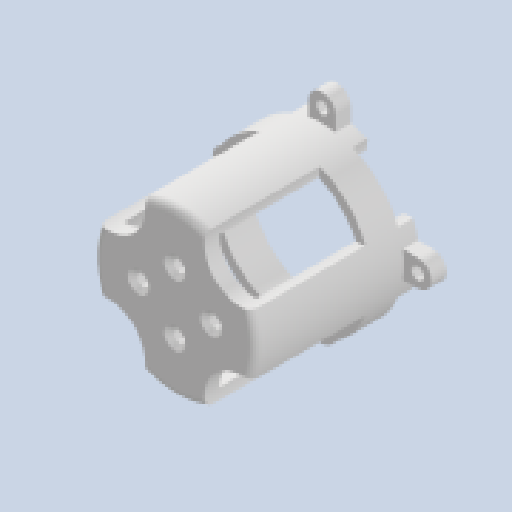
# Autodesk Inventor part: Capac_MOTOR
Saved by Autodesk Inventor 2024 (Build 280153000, 153)
## iProperties
Created: 2024-04-22
Part Number: Capac_MOTOR
Material: Generic
Document SubType Name: Modeling
Designer: mirun
Density: 1 g/cm^3
Appearance: Default
Author: mirun
Autodesk Inventor part; units mm, degrees
ref_plane "YZ Plane" through (0, 0, 0) normal (1, 0, 0) x (0, 1, 0)
ref_plane "XZ Plane" through (0, 0, 0) normal (0, 1, 0) x (-1, 0, 0)
sketch "Sketch1" plane through (0, 0, 0) normal (0, 0, 1) x (1, 0, 0)
  arc A0 (-3.5, -25) -> (3.5, -25) centre (0, -25) ccw
  line L0 (3.5, -25) -> (3.5, -21.1118)
  arc A1 (3.5, -21.1118) -> (21.1118, -3.5) centre (0, 0) ccw
  line L1 (21.1118, -3.5) -> (25, -3.5)
  arc A2 (25, -3.5) -> (25, 3.5) centre (25, 0) ccw
  line L2 (25, 3.5) -> (21.1118, 3.5)
  arc A3 (21.1118, 3.5) -> (3.5, 21.1118) centre (0, 0) ccw
  line L3 (3.5, 21.1118) -> (3.5, 25)
  arc A4 (3.5, 25) -> (-3.5, 25) centre (0, 25) ccw
  line L4 (-3.5, 25) -> (-3.5, 21.1118)
  arc A5 (-3.5, 21.1118) -> (-21.1118, 3.5) centre (0, 0) ccw
  line L5 (-21.1118, 3.5) -> (-25, 3.5)
  arc A6 (-25, 3.5) -> (-25, -3.5) centre (-25, 0) ccw
  line L6 (-25, -3.5) -> (-21.1118, -3.5)
  arc A7 (-21.1118, -3.5) -> (-3.5, -21.1118) centre (0, 0) ccw
  line L7 (-3.5, -21.1118) -> (-3.5, -25)
  circle A8 centre (0, -25) radius 1.5625
  circle A9 centre (25, 0) radius 1.5625
  circle A10 centre (-25, 0) radius 1.5625
  circle A11 centre (0, 25) radius 1.5625
  constraints: 16 end point, 16 point on circle, 12 centre point
extrude "Extrusion1" add sketch "Sketch1" along normal blind 4
sketch "Sketch2" plane through (0, 0, 4) normal (0, 0, 1) x (1, 0, 0)
  line L0 (-21.4, 0) -> (-21.4, -9.25) construction
  line L1 (-21.4, 0) -> (-21.4, 9.25) construction
  line L2 (-21.4, 0) -> (-14.9, 0) construction
  arc A0 (-21.4, -9.25) -> (-21.4, 9.25) centre (-24.7317, 0) ccw construction
  line L3 (0, -21.4) -> (0, -14.9) construction
  arc A1 (9.25, -21.4) -> (-9.25, -21.4) centre (0, -24.7317) ccw construction
  line L4 (0, -21.4) -> (9.25, -21.4) construction
  line L5 (0, -21.4) -> (-9.25, -21.4) construction
  line L6 (21.4, 0) -> (14.9, 0) construction
  arc A2 (21.4, 9.25) -> (21.4, -9.25) centre (24.7317, 0) ccw construction
  line L7 (21.4, 0) -> (21.4, 9.25) construction
  line L8 (21.4, 0) -> (21.4, -9.25) construction
  line L9 (0, 21.4) -> (0, 14.9) construction
  arc A3 (-9.25, 21.4) -> (9.25, 21.4) centre (0, 24.7317) ccw construction
  line L10 (0, 21.4) -> (-9.25, 21.4) construction
  line L11 (0, 21.4) -> (9.25, 21.4) construction
  line L12 (-5.4605, -24.8037) -> (-24.8037, -5.4605)
  line L13 (-15.1321, -15.1321) -> (-8.5913, -21.6728)
  line L14 (-15.1321, -15.1321) -> (-21.6728, -8.5913)
  line L15 (-15.1321, -15.1321) -> (-10.5359, -10.5359)
  arc A4 (-8.5913, -21.6728) -> (-21.6728, -8.5913) centre (-17.488, -17.488) ccw
  line L16 (15.1321, -15.1321) -> (10.5359, -10.5359)
  arc A5 (21.6728, -8.5913) -> (8.5913, -21.6728) centre (17.488, -17.488) ccw
  line L17 (15.1321, -15.1321) -> (21.6728, -8.5913)
  line L18 (15.1321, -15.1321) -> (8.5913, -21.6728)
  line L19 (15.1321, 15.1321) -> (10.5359, 10.5359)
  arc A6 (8.5913, 21.6728) -> (21.6728, 8.5913) centre (17.488, 17.488) ccw
  line L20 (15.1321, 15.1321) -> (8.5913, 21.6728)
  line L21 (15.1321, 15.1321) -> (21.6728, 8.5913)
  line L22 (-15.1321, 15.1321) -> (-10.5359, 10.5359)
  arc A7 (-21.6728, 8.5913) -> (-8.5913, 21.6728) centre (-17.488, 17.488) ccw
  line L23 (-15.1321, 15.1321) -> (-21.6728, 8.5913)
  line L24 (-15.1321, 15.1321) -> (-8.5913, 21.6728)
  circle A8 centre (0, 0) radius 18.9
  circle A9 centre (0, 0) radius 21.4
  point P0 (0, 0)
  point P1 (52.5406, 44.6743)
  point P2 (40.8001, 44.6743)
  point P3 (40.8001, 80.6047)
  point P4 (52.5406, 80.6047)
  point P5 (28.7051, 68.5098)
  point P6 (28.7051, 56.7692)
  point P7 (0, 0)
  point P8 (-17.2788, -7.6585)
  point P9 (-7.6585, -17.2788)
  point P10 (7.6585, -17.2788)
  point P11 (17.2788, -7.6585)
  point P12 (17.2788, 7.6585)
  point P13 (7.6585, 17.2788)
  point P14 (-7.6585, 17.2788)
  point P15 (-17.2788, 7.6585)
  point P16 (-19.8689, 7.9489)
  point P17 (-19.8689, -7.9489)
  point P18 (7.9489, 19.8689)
  point P19 (-7.9489, 19.8689)
  point P20 (19.8689, -7.9489)
  point P21 (19.8689, 7.9489)
  point P22 (-7.9489, -19.8689)
  point P23 (7.9489, -19.8689)
  dimension "d7" = 360
  dimension "d25" = 9.25
  dimension "d26" = 9.25
  dimension "d27" = 6.5
  dimension "d28" = 360
  dimension "d30" = 37.8
  constraints: 50 end point, 24 point on circle, 10 centre point, 2 perpendicular, 2 point on line, 1 coincident, 1 midpoint, 1 tangent, 74 other
  measures "d25" distance of L14.start L13.end
  measures "d26" distance of L14.start L14.end
  measures "d27" distance of L14.start L15.end
  measures "d30" diameter of A8
extrude "Extrusion2" cut sketch "Sketch2" against normal blind 4 contours L12 A9 A4 | A9 A4 A8 L15 | L12 A4 A9 | L15 A8 A4 A9 | A8 A4 L15 | L15 A4 A8 | A4 A8 A7 A6 A5 | A9 L18 A5 | A5 A8 L16 A9 | A9 L22 A8 A7 | A7 L23 A9 | A5 L16 A8 | A9 A5 L17 | L16 A8 A5 A9 | A8 L22 A7 | A9 A7 A8 L22 | L24 A7 A9 | A5 A8 L16 | L22 A8 A7 | A9 L19 A8 A6 | A6 L20 A9 | A9 L21 A6 | A6 A8 L19 A9 | A8 L19 A6 | A6 L19 A8
extrude "Extrusion3" add sketch "Sketch2" along normal blind 34.5 contours A4 A8 A5 A9 | A9 A7 A8 A4 | A5 A8 A6 A9 | A9 A6 A8 A7
extrude "Extrusion4" add sketch "Sketch2" along normal blind 4 from surface at 34.5 contours A4 A8 A5 A9 | A9 A7 A8 A4 | A4 A8 A7 A6 A5 | A5 A8 A6 A9 | A9 A6 A8 A7
fillet "Fillet1" radius 2 4 edges at (21.4, 0, 42.5) (0, 21.4, 42.5) (0, -21.4, 42.5) (-21.4, 0, 42.5)
sketch "Sketch3" plane through (0, -24.7317, 42.5) normal (0, 0, 1) x (1, 0, 0)
  arc A0 (-17.8229, 32.3937) -> (-17.8229, 17.0698) centre (0, 24.7317) ccw construction
  arc A1 (7.1849, 6.7112) -> (18.0205, 17.5469) centre (0, 24.7317) ccw construction
  arc A2 (18.0205, 31.9166) -> (7.1849, 42.7522) centre (0, 24.7317) ccw construction
  line L0 (0, 24.7317) -> (0, 12.0452) construction
  line L1 (0, 24.7317) -> (-44.2105, 24.7317) construction
  circle A3 centre (-9.5, 24.7317) radius 1.6
  circle A4 centre (0, 16.7317) radius 1.6
  circle A5 centre (9.5, 24.7317) radius 1.6
  circle A6 centre (0, 32.7317) radius 1.6
  point P0 (-7.1849, 42.7522)
  point P1 (-18.0205, 31.9166)
  dimension "d17" = 3.2
  dimension "d18" = 9.5
  dimension "d19" = 3.2
  dimension "d20" = 8
  constraints: 4 centre point, 4 end point, 2 point on line, 2 symmetric about line, 1 horizontal, 1 vertical, 2 other
  measures "d17" diameter of A3
  measures "d18" distance of A0.centre A3.centre
  measures "d19" diameter of A4
  measures "d20" distance of A4.centre A1.centre
extrude "Extrusion5" cut sketch "Sketch3" against normal blind 36
chamfer "Chamfer1" distance 1.2 angle 45 4 edges at (-1.6, 8, 42.5) (7.9, 0, 42.5) (-1.6, -8, 42.5) (-11.1, 0, 42.5)
ref_plane "Work Plane1" through (-28.5462, -28.5462, 0) normal (0, 0, 1) x (1, 0.0000309, 0)
extrude "Extrusion6" add sketch "Sketch2" along normal blind 8.5 from surface at -4 contours A9 A4 A8 L15 | L15 A8 A4 A9 | A5 A8 L16 A9 | A9 L22 A8 A7 | L16 A8 A5 A9 | A9 A7 A8 L22 | A9 L19 A8 A6 | A6 A8 L19 A9
body "Solid1"
